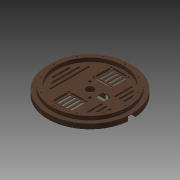
# Autodesk Inventor part: Hotplate Bottom 01
Saved by Autodesk Inventor 2015 (Build 190159000, 159)
## iProperties
Created: 2016-08-08
Part Number: Hotplate Bottom 01
Material: Generic
Document SubType Name: Modeling
Designer: spichelh
Density: 1 g/cm^3
Appearance: Default
Author: spichelh
Autodesk Inventor part; units mm, degrees
ref_plane "YZ Plane" through (0, 0, 0) normal (1, 0, 0) x (0, 1, 0)
ref_plane "XZ Plane" through (0, 0, 0) normal (0, 1, 0) x (-1, 0, 0)
ref_plane "XY Plane" through (0, 0, 0) normal (0, 0, 1) x (1, 0, 0)
sketch "Sketch1" plane through (0, 0, 0) normal (0, 1, 0) x (-1, 0, 0)
  circle A0 centre (0, 0) radius 77.5
  dimension "d0" = 155
  constraints: 1 centre point, 1 coincident
  measures "d0" diameter of A0
extrude "Extrusion1" add sketch "Sketch1" along normal blind 16
sketch "Sketch2" plane through (0, 16, 0) normal (0, 1, 0) x (1, 0, 0)
  circle A0 centre (0, 0) radius 62
  circle A1 centre (0, 0) radius 70
  circle A2 centre (0, 0) radius 77.5 projected
  dimension "d3" = 140
  dimension "d4" = 124
  constraints: 2 centre point, 2 coincident
  measures "d3" diameter of A1
  measures "d4" diameter of A0
extrude "Extrusion2" cut sketch "Sketch2" against normal blind 7
sketch "Sketch3" plane through (0, 9, 0) normal (0, 1, 0) x (1, 0, 0)
  circle A0 centre (0, 0) radius 10
  dimension "d7" = 20
  constraints: 1 centre point, 1 coincident
  measures "d7" diameter of A0
extrude "Extrusion3" [suppressed]
sketch "Sketch4" plane through (0, 0, 0) normal (0, -1, 0) x (1, 0, 0)
  circle A0 centre (0, 0) radius 67.3336 construction
  line L0 (0, 0) -> (-67.3336, 0) construction
  line L1 (0, 0) -> (0, 67.3336) construction
  line L2 (0, 0) -> (67.3336, 0) construction
  line L3 (0, 0) -> (0, -67.3336) construction
  line L4 (0, 0) -> (47.612, 47.612) construction
  circle A1 centre (0, 0) radius 77.5 construction
  line L5 (0, 0) -> (67.3336, 0) construction
  line L6 (0, 0) -> (-47.612, 47.612) construction
  line L7 (0, 0) -> (-47.612, -47.612) construction
  line L8 (0, 0) -> (47.612, -47.612) construction
  point P0 (-67.3336, 0)
  point P1 (0, -67.3336)
  point P2 (67.3336, 0)
  point P3 (47.612, -47.612)
  point P4 (47.612, 47.612)
  point P5 (-47.612, 47.612)
  point P6 (-47.612, -47.612)
  dimension "d49" = 45
  dimension "d52" = 360
  constraints: 20 end point, 4 point on line, 3 horizontal, 2 coincident, 1 equal length, 1 perpendicular, 1 vertical, 27 other
  measures "d49" angle of L5 L4
sketch "Sketch5" plane through (0, 16, 0) normal (0, 1, 0) x (1, 0, 0)
  line L0 (0, 0) -> (-36.6714, 0) construction
  circle A0 centre (-66, 0) radius 1.5
  circle A1 centre (0, 0) radius 70 construction
  circle A2 centre (0, 0) radius 62 construction
  circle A3 centre (-57.1577, -33) radius 1.5
  circle A4 centre (-33, -57.1577) radius 1.5
  circle A5 centre (0, -66) radius 1.5
  circle A6 centre (33, -57.1577) radius 1.5
  circle A7 centre (57.1577, -33) radius 1.5
  circle A8 centre (66, 0) radius 1.5
  circle A9 centre (57.1577, 33) radius 1.5
  circle A10 centre (33, 57.1577) radius 1.5
  circle A11 centre (0, 66) radius 1.5
  circle A12 centre (-33, 57.1577) radius 1.5
  circle A13 centre (-57.1577, 33) radius 1.5
  dimension "d10" = 3
  dimension "d11" = 132
  dimension "d14" = 360
  constraints: 12 centre point, 2 end point, 1 horizontal, 1 point on line, 25 other
  measures "d10" diameter of A0
  measures "d11" diameter of A0.centre A2.centre
extrude "Extrusion4" cut sketch "Sketch5" against normal blind 1.5
fillet "Fillet1" radius 1.5 12 edges at (-34.5, 14.5, -57.1577) (-1.5, 14.5, -66) (31.5, 14.5, -57.1577) (55.6577, 14.5, -33) (-58.6577, 14.5, -33) (-67.5, 14.5, 0) (-58.6577, 14.5, 33) (-34.5, 14.5, 57.1577) (-1.5, 14.5, 66) (31.5, 14.5, 57.1577) (55.6577, 14.5, 33) (64.5, 14.5, 0)
sketch "Sketch6" plane through (0, 0, 0) normal (0, -1, 0) x (1, 0, 0)
  line L0 (-19, 60) -> (19, 60)
  line L1 (21, 58) -> (21, 20)
  line L2 (19, 18) -> (-19, 18)
  line L3 (-21, 20) -> (-21, 58)
  line L4 (0, 0) -> (85.6129, 0) construction
  arc A0 (-19, 60) -> (-21, 58) centre (-19, 58) ccw
  arc A1 (-21, 20) -> (-19, 18) centre (-19, 20) ccw
  arc A2 (19, 18) -> (21, 20) centre (19, 20) ccw
  arc A3 (21, 58) -> (19, 60) centre (19, 58) ccw
  line L5 (-19, -60) -> (19, -60)
  line L6 (21, -58) -> (21, -20)
  line L7 (19, -18) -> (-19, -18)
  line L8 (-21, -20) -> (-21, -58)
  arc A4 (-21, -58) -> (-19, -60) centre (-19, -58) ccw
  arc A5 (-19, -18) -> (-21, -20) centre (-19, -20) ccw
  arc A6 (21, -20) -> (19, -18) centre (19, -20) ccw
  arc A7 (19, -60) -> (21, -58) centre (19, -58) ccw
  point P0 (-21, 60)
  point P1 (21, 18)
  point P2 (21, 60)
  point P3 (-21, -60)
  point P4 (21, -18)
  point P5 (21, -60)
  dimension "d19" = 42
  dimension "d20" = 42
  dimension "d21" = 18
  dimension "d22" = 21
  dimension "d23" = 2
  constraints: 18 end point, 16 point on circle, 15 symmetric about line, 12 point on line, 8 centre point, 8 tangent, 3 equal radius, 2 horizontal, 2 parallel, 1 perpendicular, 4 other
  measures "d19" distance of point (-21, 60) point (21, 60)
  measures "d20" distance of point (21, 60) point (21, 18)
  measures "d21" distance from line of L4.start L2
  measures "d22" distance from line of L4.start L3
  measures "d23" radius of A0
extrude "Extrusion5" cut sketch "Sketch6" against normal blind 8
sketch "Sketch7" plane through (0, 8, 0) normal (0, -1, 0) x (1, 0, 0)
  line L0 (-15, 52) -> (-15, 26) construction
  line L1 (-17, 50) -> (-17, 28)
  line L2 (-13, 28) -> (-13, 50)
  arc A0 (-13, 50) -> (-17, 50) centre (-15, 50) ccw
  arc A1 (-17, 28) -> (-13, 28) centre (-15, 28) ccw
  line L3 (-21, 20) -> (-21, 58) projected
  arc A2 (-21, 20) -> (-19, 18) centre (-19, 20) ccw projected
  line L4 (19, 18) -> (-19, 18) projected
  arc A3 (19, 18) -> (21, 20) centre (19, 20) ccw projected
  line L5 (21, 58) -> (21, 20) projected
  arc A4 (21, 58) -> (19, 60) centre (19, 58) ccw projected
  line L6 (-19, 60) -> (19, 60) projected
  arc A5 (-19, 60) -> (-21, 58) centre (-19, 58) ccw projected
  line L7 (-7.5, 52) -> (-7.5, 26) construction
  line L8 (-9.5, 50) -> (-9.5, 28)
  line L9 (-5.5, 28) -> (-5.5, 50)
  arc A6 (-5.5, 50) -> (-9.5, 50) centre (-7.5, 50) ccw
  arc A7 (-9.5, 28) -> (-5.5, 28) centre (-7.5, 28) ccw
  line L10 (0, 52) -> (0, 26) construction
  line L11 (-2, 50) -> (-2, 28)
  line L12 (2, 28) -> (2, 50)
  arc A8 (2, 50) -> (-2, 50) centre (0, 50) ccw
  arc A9 (-2, 28) -> (2, 28) centre (0, 28) ccw
  line L13 (7.5, 52) -> (7.5, 26) construction
  line L14 (5.5, 50) -> (5.5, 28)
  line L15 (9.5, 28) -> (9.5, 50)
  arc A10 (9.5, 50) -> (5.5, 50) centre (7.5, 50) ccw
  arc A11 (5.5, 28) -> (9.5, 28) centre (7.5, 28) ccw
  line L16 (15, 52) -> (15, 26) construction
  line L17 (13, 50) -> (13, 28)
  line L18 (17, 28) -> (17, 50)
  arc A12 (17, 50) -> (13, 50) centre (15, 50) ccw
  arc A13 (13, 28) -> (17, 28) centre (15, 28) ccw
  line L19 (0, 0) -> (39.7996, 0)
  line L20 (-15, -52) -> (-15, -26) construction
  line L21 (-17, -50) -> (-17, -28)
  line L22 (-13, -28) -> (-13, -50)
  arc A14 (-17, -50) -> (-13, -50) centre (-15, -50) ccw
  arc A15 (-13, -28) -> (-17, -28) centre (-15, -28) ccw
  arc A16 (-5.5, -28) -> (-9.5, -28) centre (-7.5, -28) ccw
  line L23 (-5.5, -28) -> (-5.5, -50)
  line L24 (-9.5, -50) -> (-9.5, -28)
  line L25 (-7.5, -52) -> (-7.5, -26) construction
  arc A17 (-9.5, -50) -> (-5.5, -50) centre (-7.5, -50) ccw
  arc A18 (2, -28) -> (-2, -28) centre (0, -28) ccw
  line L26 (2, -28) -> (2, -50)
  line L27 (-2, -50) -> (-2, -28)
  line L28 (0, -52) -> (0, -26) construction
  arc A19 (-2, -50) -> (2, -50) centre (0, -50) ccw
  arc A20 (9.5, -28) -> (5.5, -28) centre (7.5, -28) ccw
  line L29 (9.5, -28) -> (9.5, -50)
  line L30 (5.5, -50) -> (5.5, -28)
  line L31 (7.5, -52) -> (7.5, -26) construction
  arc A21 (5.5, -50) -> (9.5, -50) centre (7.5, -50) ccw
  arc A22 (17, -28) -> (13, -28) centre (15, -28) ccw
  line L32 (17, -28) -> (17, -50)
  line L33 (13, -50) -> (13, -28)
  line L34 (15, -52) -> (15, -26) construction
  arc A23 (13, -50) -> (17, -50) centre (15, -50) ccw
  circle A24 centre (16, 55) radius 1.75
  circle A25 centre (-16, 55) radius 1.75
  circle A26 centre (16, 23) radius 1.75
  circle A27 centre (-16, 23) radius 1.75
  line L35 (16, 55) -> (-16.5426, 55) construction
  line L36 (16, 55) -> (16, 22.241) construction
  line L37 (16, 23) -> (-19, 23) construction
  arc A28 (-21, 20) -> (-19, 18) centre (-19, 20) ccw construction
  line L38 (-21, 20) -> (-21, 58) construction
  arc A29 (-19, 60) -> (-21, 58) centre (-19, 58) ccw construction
  line L39 (-19, 60) -> (19, 60) construction
  arc A30 (21, 58) -> (19, 60) centre (19, 58) ccw construction
  line L40 (21, 58) -> (21, 20) construction
  arc A31 (19, 18) -> (21, 20) centre (19, 20) ccw construction
  line L41 (19, 18) -> (-19, 18) construction
  arc A32 (19, -60) -> (21, -58) centre (19, -58) ccw construction
  line L42 (19, -60) -> (-19, -60) construction
  arc A33 (-21, -58) -> (-19, -60) centre (-19, -58) ccw construction
  line L43 (-21, -58) -> (-21, -20) construction
  arc A34 (-19, -18) -> (-21, -20) centre (-19, -20) ccw construction
  line L44 (-19, -18) -> (19, -18) construction
  arc A35 (21, -20) -> (19, -18) centre (19, -20) ccw construction
  line L45 (21, -20) -> (21, -58) construction
  circle A36 centre (0, 0) radius 77.5 construction
  line L46 (12.5, 55) -> (-12.5, 55) construction
  line L47 (11, 56.5) -> (-11, 56.5)
  line L48 (-11, 53.5) -> (11, 53.5)
  arc A37 (11, 53.5) -> (11, 56.5) centre (11, 55) ccw
  arc A38 (-11, 56.5) -> (-11, 53.5) centre (-11, 55) ccw
  line L49 (0, 39) -> (15, 39) construction
  line L50 (12.5, 23) -> (-12.5, 23) construction
  line L51 (11, 21.5) -> (-11, 21.5)
  line L52 (-11, 24.5) -> (11, 24.5)
  arc A39 (11, 21.5) -> (11, 24.5) centre (11, 23) ccw
  arc A40 (-11, 24.5) -> (-11, 21.5) centre (-11, 23) ccw
  circle A41 centre (16, -55) radius 1.75
  circle A42 centre (-16, -55) radius 1.75
  circle A43 centre (16, -23) radius 1.75
  circle A44 centre (-16, -23) radius 1.75
  line L53 (11, -56.5) -> (-11, -56.5)
  line L54 (-11, -53.5) -> (11, -53.5)
  arc A45 (11, -56.5) -> (11, -53.5) centre (11, -55) ccw
  arc A46 (-11, -53.5) -> (-11, -56.5) centre (-11, -55) ccw
  line L55 (-11, -24.5) -> (11, -24.5)
  line L56 (12.5, -23) -> (-12.5, -23) construction
  arc A47 (-11, -21.5) -> (-11, -24.5) centre (-11, -23) ccw
  line L57 (11, -21.5) -> (-11, -21.5)
  arc A48 (11, -24.5) -> (11, -21.5) centre (11, -23) ccw
  point P0 (-15, 39)
  point P1 (-7.5, 39)
  point P2 (7.5, 39)
  point P3 (-15, -39)
  point P4 (-7.5, -39)
  point P5 (0, -39)
  point P6 (7.5, -39)
  point P7 (15, -39)
  point P8 (0, 55)
  point P9 (0, 23)
  point P10 (0, -23)
  dimension "d26" = 4
  dimension "d27" = 22
  dimension "d28" = 8
  dimension "d29" = 8
  dimension "d30" = 4
  dimension "d33" = 7.5
  dimension "d95" = 3.5
  dimension "d96" = 3.5
  dimension "d97" = 32
  dimension "d98" = 3.5
  dimension "d99" = 3.5
  dimension "d100" = 32
  dimension "d101" = 5
  dimension "d102" = 5
  dimension "d103" = 32
  dimension "d104" = 5
  dimension "d105" = 3
  dimension "d106" = 22
  constraints: 118 end point, 82 point on circle, 73 symmetric about line, 36 centre point, 32 point on line, 8 tangent, 5 horizontal, 2 midpoint, 2 parallel, 2 vertical, 76 other
  measures "d26" distance between parallel lines of L1 L2
  measures "d27" distance of A1.centre A0.centre
  measures "d28" distance from line of L0.start L6
  measures "d29" distance from line of L4 L0.end
  measures "d30" distance between parallel lines of L3 L1
  measures "d33" distance of L0.end L7.end
  measures "d95" diameter of A24
  measures "d96" diameter of A25
  measures "d97" distance of A25.centre L35.start
  measures "d98" diameter of A26
  measures "d99" diameter of A27
  measures "d100" distance of L35.start L37.start
  measures "d101" distance from line of L5 L35.start
  measures "d102" distance from line of L6 L35.start
  measures "d103" distance of L37.start A27.centre
  measures "d104" distance from line of L4 A27.centre
  measures "d105" diameter of A38
  measures "d106" distance of A38.centre A37.centre
extrude "Extrusion6" cut sketch "Sketch7" against normal blind 8 contours A0 L2 A1 L1 | A6 L9 A7 L8 | A8 L12 A9 L11 | A10 L15 A11 L14 | A12 L18 A13 L17 | L21 A15 L22 A14 | L23 A17 L24 A16 | L26 A19 L27 A18 | L29 A21 L30 A20 | L32 A23 L33 A22 | A24 | A25 | A26 | A27 | A37 L48 A38 L47 | L51 A40 L52 A39 | A41 | A42 | A43 | A44 | L53 A46 L54 A45 | A47 L57 A48 L55
sketch "Sketch8" plane through (0, 0, 0) normal (0, -1, 0) x (1, 0, 0)
  circle A0 centre (0, 0) radius 7
  dimension "d40" = 14
  constraints: 1 centre point, 1 coincident
  measures "d40" diameter of A0
extrude "Extrusion7" cut sketch "Sketch8" against normal blind 15
sketch "Sketch9" plane through (0, 0, 0) normal (0, -1, 0) x (1, 0, 0)
  circle A0 centre (0, 0) radius 7 projected
  arc A1 (-21, 20) -> (-19, 18) centre (-19, 20) ccw projected
  line L0 (-21, 20) -> (-21, 58) projected
  arc A2 (-19, 60) -> (-21, 58) centre (-19, 58) ccw projected
  line L1 (-19, 60) -> (19, 60) projected
  arc A3 (21, 58) -> (19, 60) centre (19, 58) ccw projected
  line L2 (21, 58) -> (21, 20) projected
  arc A4 (19, 18) -> (21, 20) centre (19, 20) ccw projected
  line L3 (19, 18) -> (-19, 18) projected
  arc A5 (19, -60) -> (21, -58) centre (19, -58) ccw projected
  line L4 (19, -60) -> (-19, -60) projected
  arc A6 (-21, -58) -> (-19, -60) centre (-19, -58) ccw projected
  line L5 (-21, -58) -> (-21, -20) projected
  arc A7 (-19, -18) -> (-21, -20) centre (-19, -20) ccw projected
  line L6 (-19, -18) -> (19, -18) projected
  arc A8 (21, -20) -> (19, -18) centre (19, -20) ccw projected
  line L7 (21, -20) -> (21, -58) projected
  circle A9 centre (0, 0) radius 77.5 projected
  circle A10 centre (0, 0) radius 7 projected
  line L8 (0, 7) -> (93.682, 7)
  line L9 (93.682, 7) -> (93.682, -7)
  line L10 (0, -7) -> (0, 7)
  line L11 (19, 18) -> (-19, 18) projected
  line L12 (-16, 18) -> (-3.8477, 5.8477)
  line L13 (-16, 18) -> (-0.4061, 18) construction
  line L14 (-11, 18) -> (0, 7)
  line L15 (-11, 18) -> (2.8135, 18) construction
  arc A11 (0, 7) -> (0, 7) centre (0, 0) ccw
  arc A12 (-3.8477, 5.8477) -> (0, -7) centre (0, 0) ccw
  line L16 (-11, 18) -> (-16, 18)
  line L17 (-19, -18) -> (19, -18) projected
  line L18 (11, -18) -> (22, -7)
  line L19 (11, -18) -> (26.5563, -18) construction
  line L20 (16, -18) -> (27, -7)
  line L21 (16, -18) -> (31.5563, -18) construction
  line L22 (93.682, -7) -> (27, -7)
  line L23 (22, -7) -> (0, -7)
  line L24 (11, -18) -> (16, -18)
  dimension "d43" = 45
  dimension "d44" = 45
  dimension "d45" = 5
  dimension "d46" = 5
  dimension "d54" = 93.682
  dimension "d55" = 45
  dimension "d56" = 45
  dimension "d57" = 5
  dimension "d58" = 5
  constraints: 30 end point, 7 point on circle, 5 horizontal, 4 point on line, 3 parallel, 2 centre point, 2 collinear, 2 equal length, 2 tangent, 1 coincident, 1 midpoint, 1 perpendicular, 1 vertical alignment, 1 other
  measures "d43" angle of L12 L13
  measures "d44" angle of L14 L15
  measures "d45" distance of L12.start L14.start
  measures "d46" distance from line of L0 L12.start
  measures "d54" distance from line of L9 A9.centre
  measures "d55" angle of L19 L18
  measures "d56" angle of L21 L20
  measures "d57" distance of L20.start L18.start
  measures "d58" distance from line of L7 L20.start
extrude "Extrusion8" cut sketch "Sketch9" against normal blind 8 contours A0 L10 | A0 L8 A9 L22 L20 L6 L18 L23 | L10 A0 | A0 L12 L3 L14 | L8 L9 L22 A9
sketch "Sketch10" plane through (0, 0, 0) normal (0, -1, 0) x (1, 0, 0)
  line L0 (-37.5, 36.5) -> (-37.5, -36.5) construction
  line L1 (-39, 35) -> (-39, -35)
  line L2 (-36, -35) -> (-36, 35)
  arc A0 (-36, 35) -> (-39, 35) centre (-37.5, 35) ccw
  arc A1 (-39, -35) -> (-36, -35) centre (-37.5, -35) ccw
  line L3 (-21, 20) -> (-21, 58) projected
  line L4 (0, 0) -> (-86.2158, 0)
  line L5 (34.5, 44) -> (34.5, 11) construction
  line L6 (33, 42.5) -> (33, 12.5)
  line L7 (36, 12.5) -> (36, 42.5)
  arc A2 (36, 42.5) -> (33, 42.5) centre (34.5, 42.5) ccw
  arc A3 (33, 12.5) -> (36, 12.5) centre (34.5, 12.5) ccw
  line L8 (21, 58) -> (21, 20) projected
  line L9 (34.5, -44) -> (34.5, -11) construction
  line L10 (33, -42.5) -> (33, -12.5)
  line L11 (36, -12.5) -> (36, -42.5)
  arc A4 (33, -42.5) -> (36, -42.5) centre (34.5, -42.5) ccw
  arc A5 (36, -12.5) -> (33, -12.5) centre (34.5, -12.5) ccw
  line L12 (-45.5, 26.5) -> (-45.5, -26.5) construction
  line L13 (-47, 25) -> (-47, -25)
  line L14 (-44, -25) -> (-44, 25)
  arc A6 (-44, 25) -> (-47, 25) centre (-45.5, 25) ccw
  arc A7 (-47, -25) -> (-44, -25) centre (-45.5, -25) ccw
  line L15 (-53.5, 16.5) -> (-53.5, -16.5) construction
  line L16 (-55, 15) -> (-55, -15)
  line L17 (-52, -15) -> (-52, 15)
  arc A8 (-52, 15) -> (-55, 15) centre (-53.5, 15) ccw
  arc A9 (-55, -15) -> (-52, -15) centre (-53.5, -15) ccw
  line L18 (42.5, 39) -> (42.5, 11) construction
  line L19 (41, 37.5) -> (41, 12.5)
  line L20 (44, 12.5) -> (44, 37.5)
  arc A10 (44, 37.5) -> (41, 37.5) centre (42.5, 37.5) ccw
  arc A11 (41, 12.5) -> (44, 12.5) centre (42.5, 12.5) ccw
  line L21 (50.5, 34) -> (50.5, 11) construction
  line L22 (49, 32.5) -> (49, 12.5)
  line L23 (52, 12.5) -> (52, 32.5)
  arc A12 (52, 32.5) -> (49, 32.5) centre (50.5, 32.5) ccw
  arc A13 (49, 12.5) -> (52, 12.5) centre (50.5, 12.5) ccw
  line L24 (34.5, 12.5) -> (97.2684, 12.5) construction
  line L25 (34.5, 12.5) -> (97.2684, 12.5) construction
  line L26 (42.5, -39) -> (42.5, -11) construction
  line L27 (41, -37.5) -> (41, -12.5)
  line L28 (44, -12.5) -> (44, -37.5)
  arc A14 (41, -37.5) -> (44, -37.5) centre (42.5, -37.5) ccw
  arc A15 (44, -12.5) -> (41, -12.5) centre (42.5, -12.5) ccw
  line L29 (50.5, -34) -> (50.5, -11) construction
  line L30 (49, -32.5) -> (49, -12.5)
  line L31 (52, -12.5) -> (52, -32.5)
  arc A16 (49, -32.5) -> (52, -32.5) centre (50.5, -32.5) ccw
  arc A17 (52, -12.5) -> (49, -12.5) centre (50.5, -12.5) ccw
  point P0 (-37.5, 0)
  point P1 (34.5, 27.5)
  point P2 (34.5, -27.5)
  point P3 (-45.5, 0)
  point P4 (-53.5, 0)
  point P5 (42.5, 25)
  point P6 (50.5, 22.5)
  point P7 (42.5, -25)
  point P8 (50.5, -22.5)
  dimension "d59" = 3
  dimension "d60" = 15
  dimension "d61" = 70
  dimension "d62" = 3
  dimension "d72" = 12
  dimension "d73" = 30
  dimension "d74" = 25
  dimension "d75" = 3
  dimension "d76" = 3
  dimension "d77" = 8
  dimension "d78" = 8
  dimension "d79" = 50
  dimension "d80" = 30
  dimension "d81" = 3
  dimension "d82" = 3
  dimension "d83" = 8
  dimension "d84" = 8
  dimension "d85" = 25
  dimension "d86" = 20
  dimension "d87" = 0
  constraints: 78 end point, 54 point on circle, 27 symmetric about line, 24 tangent, 23 point on line, 18 centre point, 8 parallel, 6 midpoint, 4 vertical, 2 horizontal, 1 collinear, 6 other
  measures "d59" diameter of A1
  measures "d60" distance between parallel lines of L3 L2
  measures "d61" distance of A1.centre A0.centre
  measures "d62" diameter of A3
  measures "d72" distance between parallel lines of L6 L8
  measures "d73" distance of L24.start A2.centre
  measures "d74" diameter of L24.start L4
  measures "d75" diameter of A7
  measures "d76" diameter of A9
  measures "d77" distance between parallel lines of L12 L0
  measures "d78" distance between parallel lines of L15 L12
  measures "d79" distance of A7.centre A6.centre
  measures "d80" distance of A9.centre A8.centre
  measures "d81" diameter of A11
  measures "d82" diameter of A13
  measures "d83" distance between parallel lines of L5 L18
  measures "d84" distance between parallel lines of L21 L18
  measures "d85" distance of A11.centre A10.centre
  measures "d86" distance of A13.centre A12.centre
  measures "d87" distance between parallel lines of L24 L25
extrude "Extrusion9" cut sketch "Sketch10" against normal blind 12
sketch "Sketch11" plane through (0, 9, 0) normal (0, 1, 0) x (1, 0, 0)
  line L0 (-16.5307, 16.5307) -> (14.9619, -14.9619) construction
  line L1 (0, 0) -> (0, 17.3361) construction
  circle A0 centre (-12.9047, 12.9047) radius 2.6
  circle A1 centre (12.9047, -12.9047) radius 2.6
  dimension "d88" = 45
  dimension "d89" = 5.2
  dimension "d90" = 5.2
  dimension "d91" = 18.25
  dimension "d92" = 18.25
  constraints: 4 end point, 3 point on line, 2 centre point, 1 vertical
  measures "d88" angle of L1 L0
  measures "d89" diameter of A0
  measures "d90" diameter of A1
  measures "d91" distance of L1.start A1.centre
  measures "d92" distance of L1.start A0.centre
extrude "Extrusion10" cut sketch "Sketch11" against normal blind 12
sketch "Sketch12" plane through (0, 8, 0) normal (0, -1, 0) x (1, 0, 0)
  arc A0 (13, -50) -> (17, -50) centre (15, -50) ccw projected
  line L0 (13, -50) -> (13, -28) projected
  arc A1 (17, -28) -> (13, -28) centre (15, -28) ccw projected
  line L1 (17, -28) -> (17, -50) projected
  arc A2 (-5.5, -28) -> (-9.5, -28) centre (-7.5, -28) ccw projected
  line L2 (-5.5, -28) -> (-5.5, -50) projected
  arc A3 (-9.5, -50) -> (-5.5, -50) centre (-7.5, -50) ccw projected
  line L3 (-9.5, -50) -> (-9.5, -28) projected
  arc A4 (-17, -50) -> (-13, -50) centre (-15, -50) ccw projected
  line L4 (-17, -50) -> (-17, -28) projected
  arc A5 (-13, -28) -> (-17, -28) centre (-15, -28) ccw projected
  line L5 (-13, -28) -> (-13, -50) projected
  arc A6 (-11, -53.5) -> (-11, -56.5) centre (-11, -55) ccw projected
  line L6 (-11, -53.5) -> (11, -53.5) projected
  arc A7 (11, -56.5) -> (11, -53.5) centre (11, -55) ccw projected
  line L7 (11, -56.5) -> (-11, -56.5) projected
  circle A8 centre (-16, -23) radius 1.75 projected
  circle A9 centre (16, -55) radius 1.75 projected
  circle A10 centre (16, -23) radius 1.75 projected
  circle A11 centre (-16, -55) radius 1.75 projected
  arc A12 (-11, -21.5) -> (-11, -24.5) centre (-11, -23) ccw projected
  line L8 (-11, -21.5) -> (11, -21.5) projected
  arc A13 (11, -24.5) -> (11, -21.5) centre (11, -23) ccw projected
  line L9 (11, -24.5) -> (-11, -24.5) projected
  arc A14 (2, -28) -> (-2, -28) centre (0, -28) ccw projected
  line L10 (2, -28) -> (2, -50) projected
  arc A15 (-2, -50) -> (2, -50) centre (0, -50) ccw projected
  line L11 (-2, -50) -> (-2, -28) projected
  arc A16 (5.5, -50) -> (9.5, -50) centre (7.5, -50) ccw projected
  line L12 (5.5, -50) -> (5.5, -28) projected
  arc A17 (9.5, -28) -> (5.5, -28) centre (7.5, -28) ccw projected
  line L13 (9.5, -28) -> (9.5, -50) projected
  line L14 (19, -60) -> (-19, -60) projected
  arc A18 (19, -60) -> (21, -58) centre (19, -58) ccw projected
  line L15 (21, -20) -> (21, -58) projected
  arc A19 (21, -20) -> (19, -18) centre (19, -20) ccw projected
  line L16 (16, -18) -> (19, -18) projected
  line L17 (27, -7) -> (16, -18) projected
  line L18 (77.1832, -7) -> (27, -7) projected
  arc A20 (77.1832, -7) -> (77.1832, 7) centre (0, 0) ccw projected
  line L19 (0, 7) -> (77.1832, 7) projected
  arc A21 (0, -7) -> (0, 7) centre (0, 0) ccw projected
  line L20 (22, -7) -> (0, -7) projected
  line L21 (11, -18) -> (22, -7) projected
  line L22 (-19, -18) -> (11, -18) projected
  arc A22 (-19, -18) -> (-21, -20) centre (-19, -20) ccw projected
  line L23 (-21, -58) -> (-21, -20) projected
  arc A23 (-21, -58) -> (-19, -60) centre (-19, -58) ccw projected
  line L24 (19, 7) -> (30, 7)
  line L25 (32, 5) -> (32, -5)
  line L26 (30, -7) -> (19, -7)
  line L27 (17, -5) -> (17, 5)
  arc A24 (32, 5) -> (30, 7) centre (30, 5) ccw
  arc A25 (19, 7) -> (17, 5) centre (19, 5) ccw
  arc A26 (17, -5) -> (19, -7) centre (19, -5) ccw
  arc A27 (30, -7) -> (32, -5) centre (30, -5) ccw
  point P0 (17, 7)
  dimension "d107" = 17
  dimension "d108" = 2
  dimension "d111" = 15
  constraints: 8 end point, 8 point on circle, 8 tangent, 4 centre point, 4 point on line, 3 equal radius, 2 parallel, 1 horizontal, 1 perpendicular
  measures "d107" distance from line of point (0, 0) L27
  measures "d108" radius of A24
  measures "d111" distance between parallel lines of L25 L27
extrude "Extrusion11" cut sketch "Sketch12" against normal blind 12 contours L26 L20 A26 L27 A25 L19 A24 L25 A27 L18
body "Solid1"
